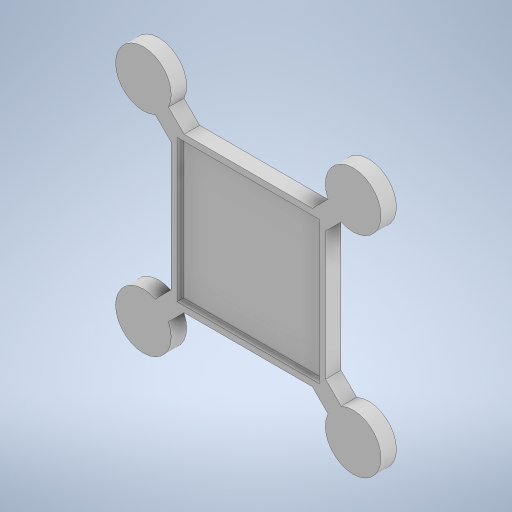
# Autodesk Inventor part: aruco_holder
Saved by Autodesk Inventor 2024 (Build 280153000, 153)
## iProperties
Created: 2023-05-06
Part Number: aruco_holder
Material: Generic
Document SubType Name: Modeling
Designer: Sujith
Density: 1 g/cm^3
Appearance: Default
Author: Sujith
Autodesk Inventor part; units mm, degrees
ref_plane "YZ Plane" through (0, 0, 0) normal (1, 0, 0) x (0, 1, 0)
ref_plane "XZ Plane" through (0, 0, 0) normal (0, 1, 0) x (-1, 0, 0)
ref_plane "XY Plane" through (0, 0, 0) normal (0, 0, 1) x (1, 0, 0)
sketch "Sketch1" plane through (0, 0, 0) normal (0, 0, 1) x (1, 0, 0)
  line L0 (-25, 25) -> (25, 25)
  line L1 (25, 25) -> (25, -25)
  line L2 (25, -25) -> (-25, -25)
  line L3 (-25, -25) -> (-25, 25)
  line L4 (-25, 25) -> (25, -25) construction
  line L5 (25, 25) -> (-25, -25) construction
  line L6 (0, 0) -> (-33.9411, 33.9411)
  circle A0 centre (-33.9411, 33.9411) radius 9
  line L7 (0, 0) -> (2.1213, 2.1213)
  line L8 (0, 0) -> (-2.1213, -2.1213)
  line L9 (2.1213, 2.1213) -> (-25.8198, 30.0624)
  line L10 (-2.1213, -2.1213) -> (-30.0624, 25.8198)
  line L11 (0, 0) -> (33.9411, -33.9411)
  circle A1 centre (33.9411, -33.9411) radius 9
  line L12 (2.1213, 2.1213) -> (30.0624, -25.8198)
  line L13 (-2.1213, -2.1213) -> (25.8198, -30.0624)
  line L14 (0, 25) -> (0, -25) construction
  line L15 (25, 25) -> (-25, 25)
  line L16 (-25, 25) -> (-25, -25)
  line L17 (-25, -25) -> (25, -25)
  line L18 (25, -25) -> (25, 25)
  line L19 (25, 25) -> (-25, -25) construction
  line L20 (-25, 25) -> (25, -25) construction
  line L21 (0, 0) -> (33.9411, 33.9411)
  circle A2 centre (33.9411, 33.9411) radius 9
  line L22 (0, 0) -> (-2.1213, 2.1213)
  line L23 (0, 0) -> (2.1213, -2.1213)
  line L24 (-2.1213, 2.1213) -> (25.8198, 30.0624)
  line L25 (2.1213, -2.1213) -> (30.0624, 25.8198)
  line L26 (0, 0) -> (-33.9411, -33.9411)
  circle A3 centre (-33.9411, -33.9411) radius 9
  line L27 (-2.1213, 2.1213) -> (-30.0624, -25.8198)
  line L28 (2.1213, -2.1213) -> (-25.8198, -30.0624)
  point P0 (-25, 20.7574)
  point P1 (-25, -20.7574)
  point P2 (-20.7574, -25)
  point P3 (20.7574, -25)
  point P4 (25, -20.7574)
  point P5 (25, 20.7574)
  point P6 (20.7574, 25)
  point P7 (-20.7574, 25)
  dimension "d0" = 50
  dimension "d1" = 50
  dimension "d5" = 48
  dimension "d6" = 18
  dimension "d7" = 3
  dimension "d8" = 3
  constraints: 58 end point, 18 symmetric about line, 8 point on circle, 4 centre point, 4 coincident, 4 midpoint, 4 point on line, 3 parallel, 1 horizontal, 1 perpendicular, 3 other
  measures "d0" distance of L1.end L2.end
  measures "d1" distance of L0.end L1.end
  measures "d5" distance of L6.start L6.end
  measures "d6" diameter of A0
  measures "d7" distance of L6.start L7.end
  measures "d8" distance of L6.start L8.end
extrude "Extrusion1" add sketch "Sketch1" along normal blind 5
sketch "Sketch2" plane through (0, 0, 5) normal (0, 0, 1) x (1, 0, 0)
  line L0 (-23, 23) -> (23, 23)
  line L1 (23, 23) -> (23, -23)
  line L2 (23, -23) -> (-23, -23)
  line L3 (-23, -23) -> (-23, 23)
  line L4 (-23, 23) -> (23, -23) construction
  line L5 (23, 23) -> (-23, -23) construction
  point P0 (0, 0)
  dimension "d11" = 46
  dimension "d12" = 46
  constraints: 12 end point, 2 midpoint, 2 parallel, 1 horizontal, 1 perpendicular
  measures "d11" distance of L1.end L2.end
  measures "d12" distance of L0.end L1.end
extrude "Extrusion2" cut sketch "Sketch2" against normal blind 2
body "Solid1"
